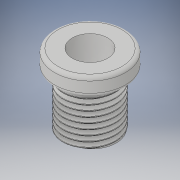
# Autodesk Inventor part: macho_m10
Saved by Autodesk Inventor 2019 (Build 230136000, 136)
## iProperties
Created: 2018-12-22
Part Number: macho_m10
Material: Generic
Document SubType Name: Modeling
Designer: assman
Density: 1 g/cm^3
Appearance: Default
Author: assman
## iProperties of the stored document macho_m10_3DPrint.ipt
Created: 2018-12-22
Part Number: macho_m10_3DPrint
Material: Generic
Document SubType Name: Modeling
Designer: assman
Density: 1 g/cm^3
Appearance: Default
Author: assman
Autodesk Inventor part; units mm, degrees
ref_plane "YZ Plane" through (0, 0, 0) normal (1, 0, 0) x (0, 1, 0)
ref_plane "XZ Plane" through (0, 0, 0) normal (0, 1, 0) x (-1, 0, 0)
ref_plane "XY Plane" through (0, 0, 0) normal (0, 0, 1) x (1, 0, 0)
sketch "Sketch1" plane through (0, 0, 0) normal (0, 1, 0) x (-1, 0, 0)
  circle A0 centre (0, 0) radius 7.5
  dimension "d0" = 15
  constraints: 1 centre point, 1 coincident
  measures "d0" diameter of A0
extrude "Extrusion1" add sketch "Sketch1" along normal blind 15
thread "Thread1" size "M15x1.5" class "6g" standard "ANSI Metric M Profile" full length
sketch "Sketch3" plane through (0, 15, 0) normal (1, 0, 0) x (0, 0, 1)
  line L0 (7.5, 0) -> (7.5, 15)
  line L1 (7.5, 15) -> (6.3878, 15)
  line L2 (6.3878, 15) -> (6.3878, 0)
  line L3 (6.3878, 0) -> (7.5, 0)
  line L4 (0, -3) -> (0, 18) projected
  constraints: 8 end point
revolve "Revolution1" cut sketch "Sketch3" angle 360 about axis through (0, 15, 0) along (0, -1, 0)
sketch "Sketch4" plane through (0, 15, 0) normal (1, 0, 0) x (0, 0, 1)
  line L0 (7.5, 0) -> (7.5, 15)
  line L1 (7.5, 15) -> (6.3878, 15)
  line L2 (6.3878, 15) -> (6.3878, 0)
  line L3 (6.3878, 0) -> (7.5, 0)
  line L4 (0, -3) -> (0, 18) projected
  constraints: 8 end point
revolve "Revolution2" add sketch "Sketch4" angle 360 about axis through (0, 15, 0) along (0, -1, 0) separate body
sketch "Sketch2" plane through (0, 15, 0) normal (-1, 0, 0) x (0, -1, 0)
  line L0 (-0.8751, -6.4638) -> (-0.7501, -6.4638) construction
  line L1 (0.1249, -7.4243) -> (-0.0001, -7.6644) construction
  line L2 (-1.5001, -7.6644) -> (-1.6251, -7.4243) construction
  line L3 (-0.6251, -6.4638) -> (-0.7501, -6.2237) construction
  line L4 (-0.7501, -6.2237) -> (-0.8751, -6.4638) construction
  line L5 (-1.5001, -7.6644) -> (-1.3751, -7.4243) construction
  line L6 (-0.6251, -6.4638) -> (-0.1251, -7.4243)
  line L7 (-1.6251, -7.4243) -> (-1.3751, -7.4243) construction
  arc A0 (-1.6251, -7.4243) -> (-1.5001, -7.5002) centre (-1.5001, -7.3592) ccw construction
  line L8 (0.1249, -7.4243) -> (-0.1251, -7.4243) construction
  line L9 (-1.5001, -7.6644) -> (-1.5001, -7.4243) construction
  line L10 (-0.0001, -7.6644) -> (-0.0001, -7.4243) construction
  line L11 (-0.7501, -6.2237) -> (-0.7501, -6.388) construction
  line L12 (-1.5001, -7.5002) -> (-0.0001, -7.5002)
  arc A1 (-1.5001, -7.5002) -> (-1.3751, -7.4243) centre (-1.5001, -7.3592) ccw
  line L13 (-0.1251, -7.4243) -> (-0.0001, -7.6644) construction
  line L14 (-1.3751, -7.4243) -> (-0.8751, -6.4638)
  line L15 (-0.0001, -0.0002) -> (-0.0001, 0.0177)
  line L16 (-0.0001, 0.0177) -> (-0.0001, -0.0002)
  line L17 (-0.0001, -0.0002) -> (0.0334, -0.0002)
  arc A2 (-0.1251, -7.4243) -> (-0.0001, -7.5002) centre (-0.0001, -7.3592) ccw
  arc A3 (-0.0001, -7.5002) -> (0.1249, -7.4243) centre (-0.0001, -7.3592) ccw construction
  arc A4 (-0.7501, -6.388) -> (-0.8751, -6.4638) centre (-0.7501, -6.5289) ccw
  arc A5 (-0.6251, -6.4638) -> (-0.7501, -6.388) centre (-0.7501, -6.5289) ccw
  line L18 (-0.7501, -6.388) -> (-0.7501, -6.4638) construction
  line L19 (-0.7501, -6.4638) -> (-0.6251, -6.4638) construction
  dimension "d5" = 55
  dimension "d6" = 0.2401
  dimension "d7" = 0.2401
  dimension "Sketch2_ThreadOffset" = 0
  dimension "Sketch2_MajorRadius" = 7.5
  dimension "d10" = 1.5
  dimension "Sketch2_MinorRadius" = 6.3878
  constraints: 40 end point, 12 point on circle, 10 parallel, 8 tangent, 6 centre point, 6 collinear, 2 midpoint, 2 point on line, 1 horizontal, 1 perpendicular, 3 other
  measures "d5" angle of L6 L14
  measures "d6" distance of L3.end L0.end
  measures "d7" distance of L1.end L10.end
  measures "Sketch2_ThreadOffset" distance between parallel lines of L15 L10
  measures "Sketch2_MajorRadius" distance from line of L12 L15.start
  measures "d10" distance from line of L1.end L9
  measures "Sketch2_MinorRadius" distance edge to line of A5 L17
coil "Coil1" sketch "Sketch2" operation cut axis through (0, 15, 0) along (0, -1, 0) pitch 1.5015 turns 11.988012 hand right bodies 2
combine bodies "Combine1" operation type add bodies to combine 1 2
sketch "Sketch5" plane through (0, 15, 0) normal (0, 1, 0) x (0.9999963, 0, -0.0027114)
  circle A0 centre (0, 0) radius 10
  dimension "d24" = 20
  constraints: 1 centre point, 1 coincident
  measures "d24" diameter of A0
extrude "Extrusion2" add sketch "Sketch5" along normal blind 5 bodies 1
fillet "Fillet1" radius 1 2 edges at (-10, 20, 0.0271) (-10, 15, 0.0271)
sketch "Sketch6" plane through (0, 20, 0) normal (0, 1, 0) x (1, 0, 0)
  circle A0 centre (0, 0) radius 5
  dimension "d28" = 10
  constraints: 1 centre point, 1 coincident
  measures "d28" diameter of A0
extrude "Extrusion3" cut sketch "Sketch6" against normal through all bodies 1
equation "\"d5\" = d12"
equation "\"d6\" = 0.160083 * Sketch2_Pitch"
equation "\"d7\" = 0.160083 * Sketch2_Pitch"
equation "\"d10\" = Sketch2_Pitch"
equation "\"d12\" = 55deg"
equation "\"Sketch2_Pitch\" = 1.5"
body "Solid1"
